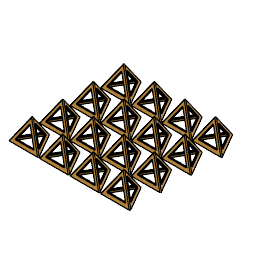
DAY 15 Painter's Tripod (Autodesk Fusion 360 design; units mm, degrees)
part number: 2026-07-31-16-48-40-662
part number: 2026-07-31-16-49-48-167
Autodesk Fusion 360 part; units mm, degrees
sketch "base profile" plane through (0, 0, 0) normal (0, 1, 0) x (1, 0, 0) in component "painter's tripod"
  line L0 (-25, -14.4338) -> (25, -14.4338)
  line L1 (25, -14.4338) -> (0, 28.8675)
  line L2 (0, 28.8675) -> (-25, -14.4338)
  line L3 (-12.5, 7.2169) -> (25, -14.4338) construction
  line L4 (12.5, 7.2169) -> (-25, -14.4338) construction
  dimension "d1" = 50
  constraint equal L0 L2
  constraint equal L0 L1
  constraint midpoint L2 L3.start
  constraint midpoint L1 L4.start
  constraint coincident L4 origin
  constraint coincident L3 origin
  constraint horizontal L0
  measures "d1" distance of L0.start L1.end
ref_plane "WorkPlane1" through (0, 40.8248, 0) normal (0, 1, 0) x (0, 0, 1) in component "painter's tripod"
sketch "loft point" plane through (0, 40.8248, 0) normal (0, 1, 0) x (1, 0, 0) in component "painter's tripod"
loft "Loft1" add profiles "base profile" section 1 section 2 point at (0, 40.8248, 0) in component "painter's tripod"
shell "Shell1" thickness 2.5 removed faces 1 at (0, 0, 0) in component "painter's tripod"
sketch "Sketch3" plane through (0, 4.5361, 12.83) normal (0, 0.333333, 0.942809) x (1, 0, 0) in component "painter's tripod"
  line L0 (-25, -4.8113) -> (25, -4.8113)
  line L1 (25, -4.8113) -> (0, 38.49)
  line L2 (0, 38.49) -> (-25, -4.8113)
  line L3 (14.6077, 1.1887) -> (0, 26.49)
  line L4 (0, 26.49) -> (-14.6077, 1.1887)
  line L5 (-14.6077, 1.1887) -> (14.6077, 1.1887)
  dimension "d5" = -6
extrude "Extrude1" cut sketch "Sketch3" against normal up to surface (2.5 mm away) contours L3 L4 L5 in component "painter's tripod"
pattern_circular "C-Pattern1" count 3 over 360 about axis through (0, 1.75, 0) along (0, 1, 0) of "Extrude1" in component "painter's tripod"
fillet "Fillet1" radius 1 3 edges at (12.5, 20.4124, 7.2169) (-12.5, 20.4124, 7.2169) (0, 20.4124, -14.4338) in component "painter's tripod"
fillet "Fillet1" radius 0.5 9 edges at (10.7679, 17.584, 2.2169) (3.4641, 17.584, -10.4338) (10.7679, 5.6569, -6.2169) (0, 5.6569, 12.4338) (-7.3038, 17.584, 8.2169) (7.3038, 17.584, 8.2169) (-3.4641, 17.584, -10.4338) (-10.7679, 17.584, 2.2169) (-10.7679, 5.6569, -6.2169) in component "painter's tripod"
fillet "Fillet2" radius 0.5 12 edges at (8.7267, 4.8235, -5.0384) (-8.7267, 4.8235, -5.0384) (0, 4.8235, 10.0767) (10.2036, 0, -5.8911) (-10.2036, 0, -5.8911) (0, 0, 11.7821) (8.7267, 16.7507, 3.3954) (1.4229, 16.7507, -9.2552) (-1.4229, 16.7507, -9.2552) (-8.7267, 16.7507, 3.3954) (-7.3038, 16.7507, 5.8599) (7.3038, 16.7507, 5.8599) in component "painter's tripod"
pattern_linear "00000000-0000-0000-0000-000000000000" [suppressed]
component "painter's tripod" placed x (1, 0, 0) y (0, 1, 0) z (0, 0, 1) at (0, 0, 0)
component "painter's tripod" placed x (1, 0, 0) y (0, 1, 0) z (0, 0, 1) at (0, 0, 50)
component "painter's tripod" placed x (1, 0, 0) y (0, 1, 0) z (0, 0, 1) at (0, 0, 100)
component "painter's tripod" placed x (1, 0, 0) y (0, 1, 0) z (0, 0, 1) at (0, 0, 150)
component "painter's tripod" placed x (1, 0, 0) y (0, 1, 0) z (0, 0, 1) at (50, 0, 0)
component "painter's tripod" placed x (1, 0, 0) y (0, 1, 0) z (0, 0, 1) at (50, 0, 50)
component "painter's tripod" placed x (1, 0, 0) y (0, 1, 0) z (0, 0, 1) at (50, 0, 100)
component "painter's tripod" placed x (1, 0, 0) y (0, 1, 0) z (0, 0, 1) at (50, 0, 150)
component "painter's tripod" placed x (1, 0, 0) y (0, 1, 0) z (0, 0, 1) at (100, 0, 0)
component "painter's tripod" placed x (1, 0, 0) y (0, 1, 0) z (0, 0, 1) at (100, 0, 50)
component "painter's tripod" placed x (1, 0, 0) y (0, 1, 0) z (0, 0, 1) at (100, 0, 100)
component "painter's tripod" placed x (1, 0, 0) y (0, 1, 0) z (0, 0, 1) at (100, 0, 150)
component "painter's tripod" placed x (1, 0, 0) y (0, 1, 0) z (0, 0, 1) at (150, 0, 0)
component "painter's tripod" placed x (1, 0, 0) y (0, 1, 0) z (0, 0, 1) at (150, 0, 50)
component "painter's tripod" placed x (1, 0, 0) y (0, 1, 0) z (0, 0, 1) at (150, 0, 100)
component "painter's tripod" placed x (1, 0, 0) y (0, 1, 0) z (0, 0, 1) at (150, 0, 150)
equation "d2 = ( d1 * sqrt(6) ) / 3"
equation "d18 = d1"
equation "d19 = d1"
